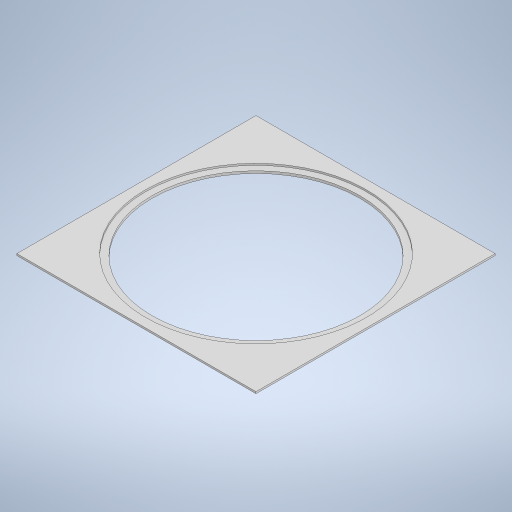
# Autodesk Inventor part: box cover
Saved by Autodesk Inventor 2024 (Build 280153000, 153)
## iProperties
Created: 2023-12-20
Part Number: box cover
Material: Generic
Document SubType Name: Modeling
Designer: 96279
Density: 1 g/cm^3
Appearance: Default
Author: 96279
Autodesk Inventor part; units mm, degrees
ref_plane "YZ Plane" through (0, 0, 0) normal (1, 0, 0) x (0, 1, 0)
ref_plane "XZ Plane" through (0, 0, 0) normal (0, 1, 0) x (-1, 0, 0)
ref_plane "XY Plane" through (0, 0, 0) normal (0, 0, 1) x (1, 0, 0)
sketch "Sketch1" plane through (0, 0, 0) normal (0, 1, 0) x (-1, 0, 0)
  line L0 (0, 0) -> (200, 0)
  line L1 (200, 0) -> (200, -200)
  line L2 (200, -200) -> (0, -200)
  line L3 (0, -200) -> (0, 0)
  circle A0 centre (100, -100) radius 92.5
  dimension "d0" = 200
  dimension "d1" = 200
  dimension "d2" = 185
  constraints: 8 end point, 2 parallel, 1 centre point, 1 horizontal, 1 perpendicular
  measures "d0" distance of L1.end L2.end
  measures "d1" distance of L0.end L1.end
  measures "d2" diameter of A0
extrude "Extrusion1" add sketch "Sketch1" against normal blind 1.5
sketch "Sketch3" plane through (0, -1.5, 0) normal (0, -1, 0) x (1, 0, 0)
  line L0 (-197.5, -2.5) -> (-2.5, -2.5)
  line L1 (-2.5, -2.5) -> (-2.5, -197.5)
  line L2 (-2.5, -197.5) -> (-197.5, -197.5)
  line L3 (-197.5, -197.5) -> (-197.5, -2.5)
  circle A0 centre (-100, -100) radius 87
  dimension "d5" = 195
  dimension "d6" = 195
  dimension "d7" = 174
  dimension "d11" = 0
  constraints: 8 end point, 2 parallel, 1 centre point, 1 horizontal, 1 perpendicular
  measures "d5" distance of L1.end L2.end
  measures "d6" distance of L0.end L1.end
  measures "d7" diameter of A0
  measures "d11" distance of A0.centre point (-100, -100)
extrude "Extrusion2" add sketch "Sketch3" along normal blind 2
body "Solid1"
